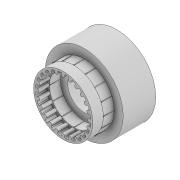
# Autodesk Inventor part: 4th Axis Barrel
Saved by Autodesk Inventor 2020 (Build 240168000, 168)
## iProperties
Created: 2021-06-26
Part Number: 4th Axis Barrel
Material: Generic
Document SubType Name: Modeling
Designer: Coy
Density: 1 g/cm^3
Appearance: Default
Author: Coy
Autodesk Inventor part; units mm, degrees
ref_plane "YZ Plane" through (0, 0, 0) normal (1, 0, 0) x (0, 1, 0)
ref_plane "XZ Plane" through (0, 0, 0) normal (0, 1, 0) x (-1, 0, 0)
ref_plane "XY Plane" through (0, 0, 0) normal (0, 0, 1) x (1, 0, 0)
sketch "Sketch1" plane through (0, 0, 0) normal (0, 0, 1) x (1, 0, 0)
  circle A0 centre (0, 0) radius 11
  circle A1 centre (0, 0) radius 26
  dimension "d0" = 22
  dimension "d1" = 52
  constraints: 2 centre point, 2 coincident
  measures "d0" diameter of A0
  measures "d1" diameter of A1
extrude "Extrusion1" add sketch "Sketch1" against normal blind 21.75
sketch "Sketch2" plane through (0, 0, 0) normal (0, 0, 1) x (1, 0, 0)
  circle A0 centre (0, 0) radius 16
  circle A1 centre (0, 0) radius 20
  dimension "d4" = 32
  dimension "d5" = 40
  constraints: 2 centre point, 2 coincident
  measures "d4" diameter of A0
  measures "d5" diameter of A1
extrude "Extrusion2" add sketch "Sketch2" along normal blind 7
chamfer "Chamfer2" distance 7 angle 2 1 edges at (-20, 0, 7) measured on face at (-20, 0, 6.5)
chamfer "Chamfer3" distance 7 angle 2 1 edges at (-16, 0, 7) measured on face at (-16, 0, 6.5)
sketch "Sketch3" plane through (0, 0, 7) normal (0, 0, 1) x (1, 0, 0)
  circle A0 centre (0, 0) radius 16 projected
  arc A1 (-0.2, 15.9988) -> (0.2, 15.9988) centre (0, 16) ccw
  circle A2 centre (0, 0) radius 16.2444 projected
  line L0 (-0.2031, 16.2432) -> (-0.2, 15.9975)
  line L1 (0.2031, 16.2432) -> (0.2, 15.9975)
  line L2 (-8.2974, 13.9655) -> (-8.1719, 13.7542)
  arc A3 (-8.1726, 13.7553) -> (-7.8262, 13.9553) centre (-8, 13.8564) ccw
  line L3 (-7.9457, 14.1685) -> (-7.8256, 13.9542)
  line L4 (-14.1685, 7.9457) -> (-13.9542, 7.8256)
  arc A4 (-13.9553, 7.8262) -> (-13.7553, 8.1726) centre (-13.8564, 8) ccw
  line L5 (-13.9655, 8.2974) -> (-13.7542, 8.1719)
  line L6 (-16.2432, -0.2031) -> (-15.9975, -0.2)
  arc A5 (-15.9988, -0.2) -> (-15.9988, 0.2) centre (-16, 0) ccw
  line L7 (-16.2432, 0.2031) -> (-15.9975, 0.2)
  line L8 (-13.9655, -8.2974) -> (-13.7542, -8.1719)
  arc A6 (-13.7553, -8.1726) -> (-13.9553, -7.8262) centre (-13.8564, -8) ccw
  line L9 (-14.1685, -7.9457) -> (-13.9542, -7.8256)
  line L10 (-7.9457, -14.1685) -> (-7.8256, -13.9542)
  arc A7 (-7.8262, -13.9553) -> (-8.1726, -13.7553) centre (-8, -13.8564) ccw
  line L11 (-8.2974, -13.9655) -> (-8.1719, -13.7542)
  line L12 (0.2031, -16.2432) -> (0.2, -15.9975)
  arc A8 (0.2, -15.9988) -> (-0.2, -15.9988) centre (0, -16) ccw
  line L13 (-0.2031, -16.2432) -> (-0.2, -15.9975)
  line L14 (8.2974, -13.9655) -> (8.1719, -13.7542)
  arc A9 (8.1726, -13.7553) -> (7.8262, -13.9553) centre (8, -13.8564) ccw
  line L15 (7.9457, -14.1685) -> (7.8256, -13.9542)
  line L16 (14.1685, -7.9457) -> (13.9542, -7.8256)
  arc A10 (13.9553, -7.8262) -> (13.7553, -8.1726) centre (13.8564, -8) ccw
  line L17 (13.9655, -8.2974) -> (13.7542, -8.1719)
  line L18 (16.2432, 0.2031) -> (15.9975, 0.2)
  arc A11 (15.9988, 0.2) -> (15.9988, -0.2) centre (16, 0) ccw
  line L19 (16.2432, -0.2031) -> (15.9975, -0.2)
  line L20 (13.9655, 8.2974) -> (13.7542, 8.1719)
  arc A12 (13.7553, 8.1726) -> (13.9553, 7.8262) centre (13.8564, 8) ccw
  line L21 (14.1685, 7.9457) -> (13.9542, 7.8256)
  line L22 (7.9457, 14.1685) -> (7.8256, 13.9542)
  arc A13 (7.8262, 13.9553) -> (8.1726, 13.7553) centre (8, 13.8564) ccw
  line L23 (8.2974, 13.9655) -> (8.1719, 13.7542)
  point P0 (-7.8262, 13.9553)
  point P1 (-13.7553, 8.1726)
  point P2 (-15.9988, 0.2)
  point P3 (-13.9553, -7.8262)
  point P4 (-8.1726, -13.7553)
  point P5 (-0.2, -15.9988)
  point P6 (7.8262, -13.9553)
  point P7 (13.7553, -8.1726)
  point P8 (15.9988, -0.2)
  point P9 (13.9553, 7.8262)
  point P10 (8.1726, 13.7553)
  point P11 (0.2, 15.9988)
  point P12 (-0.2, 15.9988)
  dimension "d17" = 0.4
  dimension "d18" = 0
  dimension "d21" = 360
  constraints: 53 point on circle, 48 end point, 12 centre point, 2 line through centre, 2 tangent, 121 other
  measures "d17" diameter of A1
  measures "d18" horizontal distance of point (0, 0) A0.start
extrude "Extrusion3" add sketch "Sketch3" against normal up to surface (7 mm away) contours A0 A11 | A0 L18 A2 L19 | A12 A0 | A0 L20 A2 L21 | L16 A2 L17 A0 | A0 A10 | A13 A0 | A0 L22 A2 L23 | L14 A2 L15 A0 | A0 A9 | A1 A0 | A0 L0 A2 L1 | L12 A2 L13 A0 | A0 A8 | A3 A0 | A0 L2 A2 L3 | L10 A2 L11 A0 | A0 A7 | A4 A0 | A0 L4 A2 L5 | L8 A2 L9 A0 | A0 A6 | A5 A0 | A0 L6 A2 L7
sketch "Sketch4" plane through (0, 0, 7) normal (0, 0, 1) x (1, 0, 0)
  circle A0 centre (0, 0) radius 20 construction
  circle A1 centre (0, 0) radius 19.7556 projected
  arc A2 (0.2, 19.999) -> (-0.2, 19.999) centre (0, 20) ccw
  line L0 (-0.2, 19.999) -> (-0.1988, 19.7546)
  line L1 (0.2, 19.999) -> (0.1988, 19.7546)
  arc A3 (-7.4685, 18.5532) -> (-7.8381, 18.4001) centre (-7.6537, 18.4776) ccw
  line L2 (-7.8381, 18.4001) -> (-7.7434, 18.1748)
  line L3 (-7.4685, 18.5532) -> (-7.3761, 18.3269)
  arc A4 (-14, 14.2828) -> (-14.2828, 14) centre (-14.1421, 14.1421) ccw
  line L4 (-14.2828, 14) -> (-14.1091, 13.828)
  line L5 (-14, 14.2828) -> (-13.828, 14.1091)
  arc A5 (-18.4001, 7.8381) -> (-18.5532, 7.4685) centre (-18.4776, 7.6537) ccw
  line L6 (-18.5532, 7.4685) -> (-18.3269, 7.3761)
  line L7 (-18.4001, 7.8381) -> (-18.1748, 7.7434)
  arc A6 (-19.999, 0.2) -> (-19.999, -0.2) centre (-20, 0) ccw
  line L8 (-19.999, -0.2) -> (-19.7546, -0.1988)
  line L9 (-19.999, 0.2) -> (-19.7546, 0.1988)
  arc A7 (-18.5532, -7.4685) -> (-18.4001, -7.8381) centre (-18.4776, -7.6537) ccw
  line L10 (-18.4001, -7.8381) -> (-18.1748, -7.7434)
  line L11 (-18.5532, -7.4685) -> (-18.3269, -7.3761)
  arc A8 (-14.2828, -14) -> (-14, -14.2828) centre (-14.1421, -14.1421) ccw
  line L12 (-14, -14.2828) -> (-13.828, -14.1091)
  line L13 (-14.2828, -14) -> (-14.1091, -13.828)
  arc A9 (-7.8381, -18.4001) -> (-7.4685, -18.5532) centre (-7.6537, -18.4776) ccw
  line L14 (-7.4685, -18.5532) -> (-7.3761, -18.3269)
  line L15 (-7.8381, -18.4001) -> (-7.7434, -18.1748)
  arc A10 (-0.2, -19.999) -> (0.2, -19.999) centre (0, -20) ccw
  line L16 (0.2, -19.999) -> (0.1988, -19.7546)
  line L17 (-0.2, -19.999) -> (-0.1988, -19.7546)
  arc A11 (7.4685, -18.5532) -> (7.8381, -18.4001) centre (7.6537, -18.4776) ccw
  line L18 (7.8381, -18.4001) -> (7.7434, -18.1748)
  line L19 (7.4685, -18.5532) -> (7.3761, -18.3269)
  arc A12 (14, -14.2828) -> (14.2828, -14) centre (14.1421, -14.1421) ccw
  line L20 (14.2828, -14) -> (14.1091, -13.828)
  line L21 (14, -14.2828) -> (13.828, -14.1091)
  arc A13 (18.4001, -7.8381) -> (18.5532, -7.4685) centre (18.4776, -7.6537) ccw
  line L22 (18.5532, -7.4685) -> (18.3269, -7.3761)
  line L23 (18.4001, -7.8381) -> (18.1748, -7.7434)
  arc A14 (19.999, -0.2) -> (19.999, 0.2) centre (20, 0) ccw
  line L24 (19.999, 0.2) -> (19.7546, 0.1988)
  line L25 (19.999, -0.2) -> (19.7546, -0.1988)
  arc A15 (18.5532, 7.4685) -> (18.4001, 7.8381) centre (18.4776, 7.6537) ccw
  line L26 (18.4001, 7.8381) -> (18.1748, 7.7434)
  line L27 (18.5532, 7.4685) -> (18.3269, 7.3761)
  arc A16 (14.2828, 14) -> (14, 14.2828) centre (14.1421, 14.1421) ccw
  line L28 (14, 14.2828) -> (13.828, 14.1091)
  line L29 (14.2828, 14) -> (14.1091, 13.828)
  arc A17 (7.8381, 18.4001) -> (7.4685, 18.5532) centre (7.6537, 18.4776) ccw
  line L30 (7.4685, 18.5532) -> (7.3761, 18.3269)
  line L31 (7.8381, 18.4001) -> (7.7434, 18.1748)
  dimension "d25" = 0.4
  dimension "d28" = 360
  constraints: 64 end point, 35 point on circle, 16 centre point, 2 tangent, 132 other
  measures "d25" diameter of A2
extrude "Extrusion4" add sketch "Sketch4" against normal up to surface (7 mm away) contours A1 L24 A14 L25 | A1 L26 A15 L27 | L22 A13 L23 A1 | A1 L28 A16 L29 | L20 A12 L21 A1 | A1 L30 A17 L31 | L18 A11 L19 A1 | A1 L0 A2 L1 | L16 A10 L17 A1 | A1 L2 A3 L3 | L14 A9 L15 A1 | A1 L4 A4 L5 | L12 A8 L13 A1 | A1 L6 A5 L7 | L10 A7 L11 A1 | A1 L8 A6 L9
sketch "Sketch5" plane through (0, 0, 7) normal (0, 0, 1) x (1, 0, 0)
  arc A0 (7.3761, 18.3269) -> (0.1988, 19.7546) centre (0, 0) ccw projected
  line L0 (-0.2031, 16.2432) -> (-0.2, 15.9987) projected
  circle A1 centre (0, 0) radius 16.2444 construction
  arc A2 (-0.1988, 19.7546) -> (-7.3761, 18.3269) centre (0, 0) ccw projected
  circle A3 centre (0, 0) radius 19.7556
  line L1 (0, 0) -> (0, 34.6201) construction
  line L2 (1.1056, 17.9252) -> (1, 16.2136) construction
  line L3 (-1.1056, 17.9252) -> (-1, 16.2136) construction
  arc A4 (-1.0636, 17.2444) -> (1.0636, 17.2444) centre (0, 17.31) ccw
  line L4 (-1.0636, 17.2444) -> (-1.1056, 17.9252)
  line L5 (1.0636, 17.2444) -> (1.1056, 17.9252)
  arc A5 (-0.2031, 16.2432) -> (-7.9457, 14.1685) centre (0, 0) ccw projected
  arc A6 (1.6859, 18.423) -> (1.1056, 17.9252) centre (1.6374, 17.8924) ccw
  arc A7 (-1.1056, 17.9252) -> (-1.6859, 18.423) centre (-1.6374, 17.8924) ccw
  arc A8 (-5.7073, 17.0283) -> (-6.3967, 17.3589) centre (-6.2125, 16.859) ccw
  line L6 (-5.4905, 16.3816) -> (-5.7073, 17.0283)
  arc A9 (-5.4905, 16.3816) -> (-3.4359, 16.9321) centre (-4.4802, 16.7202) ccw
  line L7 (-3.4359, 16.9321) -> (-3.5715, 17.6006)
  arc A10 (-3.1398, 18.2316) -> (-3.5715, 17.6006) centre (-3.0493, 17.7065) ccw
  arc A11 (-9.9201, 14.9709) -> (-10.6715, 15.1119) centre (-10.3642, 14.6766) ccw
  line L8 (-9.5433, 14.4023) -> (-9.9201, 14.9709)
  arc A12 (-9.5433, 14.4023) -> (-7.7011, 15.4659) centre (-8.655, 14.9909) ccw
  line L9 (-7.7011, 15.4659) -> (-8.0052, 16.0765)
  arc A13 (-7.7515, 16.7978) -> (-8.0052, 16.0765) centre (-7.5282, 16.314) ccw
  arc A14 (-13.4568, 11.8933) -> (-14.2192, 11.8349) centre (-13.8096, 11.4941) ccw
  line L10 (-12.9457, 11.4416) -> (-13.4568, 11.8933)
  arc A15 (-12.9457, 11.4416) -> (-11.4416, 12.9457) centre (-12.24, 12.24) ccw
  line L11 (-11.4416, 12.9457) -> (-11.8933, 13.4568)
  arc A16 (-11.8349, 14.2192) -> (-11.8933, 13.4568) centre (-11.4941, 13.8096) ccw
  arc A17 (-16.0765, 8.0052) -> (-16.7978, 7.7515) centre (-16.314, 7.5282) ccw
  line L12 (-15.4659, 7.7011) -> (-16.0765, 8.0052)
  arc A18 (-15.4659, 7.7011) -> (-14.4023, 9.5433) centre (-14.9909, 8.655) ccw
  line L13 (-14.4023, 9.5433) -> (-14.9709, 9.9201)
  arc A19 (-15.1119, 10.6715) -> (-14.9709, 9.9201) centre (-14.6766, 10.3642) ccw
  arc A20 (-17.6006, 3.5715) -> (-18.2316, 3.1398) centre (-17.7065, 3.0493) ccw
  line L14 (-16.9321, 3.4359) -> (-17.6006, 3.5715)
  arc A21 (-16.9321, 3.4359) -> (-16.3816, 5.4905) centre (-16.7202, 4.4802) ccw
  line L15 (-16.3816, 5.4905) -> (-17.0283, 5.7073)
  arc A22 (-17.3589, 6.3967) -> (-17.0283, 5.7073) centre (-16.859, 6.2125) ccw
  arc A23 (-17.9252, -1.1056) -> (-18.423, -1.6859) centre (-17.8924, -1.6374) ccw
  line L16 (-17.2444, -1.0636) -> (-17.9252, -1.1056)
  arc A24 (-17.2444, -1.0636) -> (-17.2444, 1.0636) centre (-17.31, 0) ccw
  line L17 (-17.2444, 1.0636) -> (-17.9252, 1.1056)
  arc A25 (-18.423, 1.6859) -> (-17.9252, 1.1056) centre (-17.8924, 1.6374) ccw
  arc A26 (-17.0283, -5.7073) -> (-17.3589, -6.3967) centre (-16.859, -6.2125) ccw
  line L18 (-16.3816, -5.4905) -> (-17.0283, -5.7073)
  arc A27 (-16.3816, -5.4905) -> (-16.9321, -3.4359) centre (-16.7202, -4.4802) ccw
  line L19 (-16.9321, -3.4359) -> (-17.6006, -3.5715)
  arc A28 (-18.2316, -3.1398) -> (-17.6006, -3.5715) centre (-17.7065, -3.0493) ccw
  arc A29 (-14.9709, -9.9201) -> (-15.1119, -10.6715) centre (-14.6766, -10.3642) ccw
  line L20 (-14.4023, -9.5433) -> (-14.9709, -9.9201)
  arc A30 (-14.4023, -9.5433) -> (-15.4659, -7.7011) centre (-14.9909, -8.655) ccw
  line L21 (-15.4659, -7.7011) -> (-16.0765, -8.0052)
  arc A31 (-16.7978, -7.7515) -> (-16.0765, -8.0052) centre (-16.314, -7.5282) ccw
  arc A32 (-11.8933, -13.4568) -> (-11.8349, -14.2192) centre (-11.4941, -13.8096) ccw
  line L22 (-11.4416, -12.9457) -> (-11.8933, -13.4568)
  arc A33 (-11.4416, -12.9457) -> (-12.9457, -11.4416) centre (-12.24, -12.24) ccw
  line L23 (-12.9457, -11.4416) -> (-13.4568, -11.8933)
  arc A34 (-14.2192, -11.8349) -> (-13.4568, -11.8933) centre (-13.8096, -11.4941) ccw
  arc A35 (-8.0052, -16.0765) -> (-7.7515, -16.7978) centre (-7.5282, -16.314) ccw
  line L24 (-7.7011, -15.4659) -> (-8.0052, -16.0765)
  arc A36 (-7.7011, -15.4659) -> (-9.5433, -14.4023) centre (-8.655, -14.9909) ccw
  line L25 (-9.5433, -14.4023) -> (-9.9201, -14.9709)
  arc A37 (-10.6715, -15.1119) -> (-9.9201, -14.9709) centre (-10.3642, -14.6766) ccw
  arc A38 (-3.5715, -17.6006) -> (-3.1398, -18.2316) centre (-3.0493, -17.7065) ccw
  line L26 (-3.4359, -16.9321) -> (-3.5715, -17.6006)
  arc A39 (-3.4359, -16.9321) -> (-5.4905, -16.3816) centre (-4.4802, -16.7202) ccw
  line L27 (-5.4905, -16.3816) -> (-5.7073, -17.0283)
  arc A40 (-6.3967, -17.3589) -> (-5.7073, -17.0283) centre (-6.2125, -16.859) ccw
  arc A41 (1.1056, -17.9252) -> (1.6859, -18.423) centre (1.6374, -17.8924) ccw
  line L28 (1.0636, -17.2444) -> (1.1056, -17.9252)
  arc A42 (1.0636, -17.2444) -> (-1.0636, -17.2444) centre (0, -17.31) ccw
  line L29 (-1.0636, -17.2444) -> (-1.1056, -17.9252)
  arc A43 (-1.6859, -18.423) -> (-1.1056, -17.9252) centre (-1.6374, -17.8924) ccw
  arc A44 (5.7073, -17.0283) -> (6.3967, -17.3589) centre (6.2125, -16.859) ccw
  line L30 (5.4905, -16.3816) -> (5.7073, -17.0283)
  arc A45 (5.4905, -16.3816) -> (3.4359, -16.9321) centre (4.4802, -16.7202) ccw
  line L31 (3.4359, -16.9321) -> (3.5715, -17.6006)
  arc A46 (3.1398, -18.2316) -> (3.5715, -17.6006) centre (3.0493, -17.7065) ccw
  arc A47 (9.9201, -14.9709) -> (10.6715, -15.1119) centre (10.3642, -14.6766) ccw
  line L32 (9.5433, -14.4023) -> (9.9201, -14.9709)
  arc A48 (9.5433, -14.4023) -> (7.7011, -15.4659) centre (8.655, -14.9909) ccw
  line L33 (7.7011, -15.4659) -> (8.0052, -16.0765)
  arc A49 (7.7515, -16.7978) -> (8.0052, -16.0765) centre (7.5282, -16.314) ccw
  arc A50 (13.4568, -11.8933) -> (14.2192, -11.8349) centre (13.8096, -11.4941) ccw
  line L34 (12.9457, -11.4416) -> (13.4568, -11.8933)
  arc A51 (12.9457, -11.4416) -> (11.4416, -12.9457) centre (12.24, -12.24) ccw
  line L35 (11.4416, -12.9457) -> (11.8933, -13.4568)
  arc A52 (11.8349, -14.2192) -> (11.8933, -13.4568) centre (11.4941, -13.8096) ccw
  arc A53 (16.0765, -8.0052) -> (16.7978, -7.7515) centre (16.314, -7.5282) ccw
  line L36 (15.4659, -7.7011) -> (16.0765, -8.0052)
  arc A54 (15.4659, -7.7011) -> (14.4023, -9.5433) centre (14.9909, -8.655) ccw
  line L37 (14.4023, -9.5433) -> (14.9709, -9.9201)
  arc A55 (15.1119, -10.6715) -> (14.9709, -9.9201) centre (14.6766, -10.3642) ccw
  arc A56 (17.6006, -3.5715) -> (18.2316, -3.1398) centre (17.7065, -3.0493) ccw
  line L38 (16.9321, -3.4359) -> (17.6006, -3.5715)
  arc A57 (16.9321, -3.4359) -> (16.3816, -5.4905) centre (16.7202, -4.4802) ccw
  line L39 (16.3816, -5.4905) -> (17.0283, -5.7073)
  arc A58 (17.3589, -6.3967) -> (17.0283, -5.7073) centre (16.859, -6.2125) ccw
  arc A59 (17.9252, 1.1056) -> (18.423, 1.6859) centre (17.8924, 1.6374) ccw
  line L40 (17.2444, 1.0636) -> (17.9252, 1.1056)
  arc A60 (17.2444, 1.0636) -> (17.2444, -1.0636) centre (17.31, 0) ccw
  line L41 (17.2444, -1.0636) -> (17.9252, -1.1056)
  arc A61 (18.423, -1.6859) -> (17.9252, -1.1056) centre (17.8924, -1.6374) ccw
  arc A62 (17.0283, 5.7073) -> (17.3589, 6.3967) centre (16.859, 6.2125) ccw
  line L42 (16.3816, 5.4905) -> (17.0283, 5.7073)
  arc A63 (16.3816, 5.4905) -> (16.9321, 3.4359) centre (16.7202, 4.4802) ccw
  line L43 (16.9321, 3.4359) -> (17.6006, 3.5715)
  arc A64 (18.2316, 3.1398) -> (17.6006, 3.5715) centre (17.7065, 3.0493) ccw
  arc A65 (14.9709, 9.9201) -> (15.1119, 10.6715) centre (14.6766, 10.3642) ccw
  line L44 (14.4023, 9.5433) -> (14.9709, 9.9201)
  arc A66 (14.4023, 9.5433) -> (15.4659, 7.7011) centre (14.9909, 8.655) ccw
  line L45 (15.4659, 7.7011) -> (16.0765, 8.0052)
  arc A67 (16.7978, 7.7515) -> (16.0765, 8.0052) centre (16.314, 7.5282) ccw
  arc A68 (11.8933, 13.4568) -> (11.8349, 14.2192) centre (11.4941, 13.8096) ccw
  line L46 (11.4416, 12.9457) -> (11.8933, 13.4568)
  arc A69 (11.4416, 12.9457) -> (12.9457, 11.4416) centre (12.24, 12.24) ccw
  line L47 (12.9457, 11.4416) -> (13.4568, 11.8933)
  arc A70 (14.2192, 11.8349) -> (13.4568, 11.8933) centre (13.8096, 11.4941) ccw
  arc A71 (8.0052, 16.0765) -> (7.7515, 16.7978) centre (7.5282, 16.314) ccw
  line L48 (7.7011, 15.4659) -> (8.0052, 16.0765)
  arc A72 (7.7011, 15.4659) -> (9.5433, 14.4023) centre (8.655, 14.9909) ccw
  line L49 (9.5433, 14.4023) -> (9.9201, 14.9709)
  arc A73 (10.6715, 15.1119) -> (9.9201, 14.9709) centre (10.3642, 14.6766) ccw
  arc A74 (3.5715, 17.6006) -> (3.1398, 18.2316) centre (3.0493, 17.7065) ccw
  line L50 (3.4359, 16.9321) -> (3.5715, 17.6006)
  arc A75 (3.4359, 16.9321) -> (5.4905, 16.3816) centre (4.4802, 16.7202) ccw
  line L51 (5.4905, 16.3816) -> (5.7073, 17.0283)
  arc A76 (6.3967, 17.3589) -> (5.7073, 17.0283) centre (6.2125, 16.859) ccw
  arc A77 (-1.6859, 18.423) -> (-3.1398, 18.2316) centre (0, 0) ccw
  arc A78 (-6.3967, 17.3589) -> (-7.7515, 16.7978) centre (0, 0) ccw
  arc A79 (-10.6715, 15.1119) -> (-11.8349, 14.2192) centre (0, 0) ccw
  arc A80 (-14.2192, 11.8349) -> (-15.1119, 10.6715) centre (0, 0) ccw
  arc A81 (-16.7978, 7.7515) -> (-17.3589, 6.3967) centre (0, 0) ccw
  arc A82 (-18.2316, 3.1398) -> (-18.423, 1.6859) centre (0, 0) ccw
  arc A83 (-18.423, -1.6859) -> (-18.2316, -3.1398) centre (0, 0) ccw
  arc A84 (-17.3589, -6.3967) -> (-16.7978, -7.7515) centre (0, 0) ccw
  arc A85 (-15.1119, -10.6715) -> (-14.2192, -11.8349) centre (0, 0) ccw
  arc A86 (-11.8349, -14.2192) -> (-10.6715, -15.1119) centre (0, 0) ccw
  arc A87 (-7.7515, -16.7978) -> (-6.3967, -17.3589) centre (0, 0) ccw
  arc A88 (-3.1398, -18.2316) -> (-1.6859, -18.423) centre (0, 0) ccw
  arc A89 (1.6859, -18.423) -> (3.1398, -18.2316) centre (0, 0) ccw
  arc A90 (6.3967, -17.3589) -> (7.7515, -16.7978) centre (0, 0) ccw
  arc A91 (10.6715, -15.1119) -> (11.8349, -14.2192) centre (0, 0) ccw
  arc A92 (14.2192, -11.8349) -> (15.1119, -10.6715) centre (0, 0) ccw
  arc A93 (16.7978, -7.7515) -> (17.3589, -6.3967) centre (0, 0) ccw
  arc A94 (18.2316, -3.1398) -> (18.423, -1.6859) centre (0, 0) ccw
  arc A95 (18.423, 1.6859) -> (18.2316, 3.1398) centre (0, 0) ccw
  arc A96 (17.3589, 6.3967) -> (16.7978, 7.7515) centre (0, 0) ccw
  arc A97 (15.1119, 10.6715) -> (14.2192, 11.8349) centre (0, 0) ccw
  arc A98 (11.8349, 14.2192) -> (10.6715, 15.1119) centre (0, 0) ccw
  arc A99 (7.7515, 16.7978) -> (6.3967, 17.3589) centre (0, 0) ccw
  arc A100 (3.1398, 18.2316) -> (1.6859, 18.423) centre (0, 0) ccw
  point P0 (0.1988, 19.7546)
  point P1 (-7.3761, 18.3269)
  point P2 (7.3761, 18.3269)
  dimension "d33" = 1
  dimension "d38" = 1
  dimension "d40" = 1.0656
  dimension "d41" = 1.0656
  dimension "d42" = 1.0656
  dimension "d45" = 360
  constraints: 195 point on circle, 102 end point, 97 centre point, 4 tangent, 3 coincident, 2 line through centre, 2 point on line, 1 midpoint, 1 vertical, 340 other
  measures "d33" distance from line of L1 L3.end
  measures "d38" distance from line of L1 L2.end
  measures "d40" radius of A4
  measures "d41" diameter of A7
  measures "d42" diameter of A6
extrude "Extrusion5" add sketch "Sketch5" along normal blind 7
equation "\"d41\" = d40"
equation "\"d42\" = d40"
body "Solid1"
